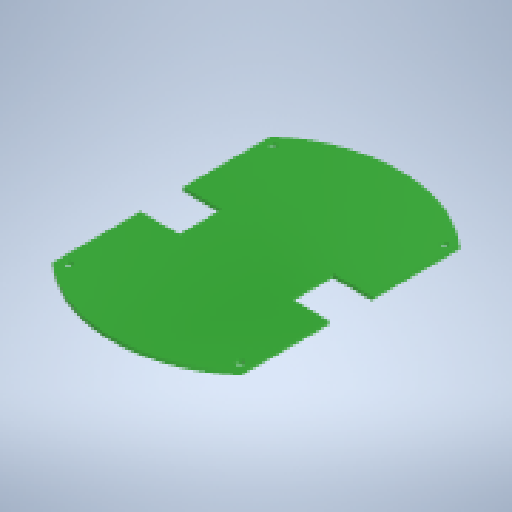
# Autodesk Inventor part: BaseBoard3
Saved by Autodesk Inventor 2025.3 (Build 293356000, 356)
## iProperties
Created: 2025-05-29
Part Number: BaseBoard3
Material: 一般
Document SubType Name: Modeling
Designer: yamashita1
Density: 1 g/cm^3
Appearance: 滑らか - 濃い深緑
Author: yamashita1
Autodesk Inventor part; units mm, degrees
ref_plane "YZ Plane" through (0, 0, 0) normal (1, 0, 0) x (0, 1, 0)
ref_plane "XZ Plane" through (0, 0, 0) normal (0, 1, 0) x (-1, 0, 0)
ref_plane "XY Plane" through (0, 0, 0) normal (0, 0, 1) x (1, 0, 0)
sketch "スケッチ1" plane through (0, 0, 0) normal (0, 0, 1) x (1, 0, 0)
  circle A0 centre (0, 0) radius 65 construction
  line L0 (-42.5, 65) -> (42.5, 65) construction
  line L1 (42.5, 65) -> (42.5, -65) construction
  line L2 (42.5, -65) -> (-42.5, -65) construction
  line L3 (-42.5, -65) -> (-42.5, 65) construction
  arc A1 (42.5, 49.1808) -> (-42.5, 49.1808) centre (0, 0) ccw
  line L4 (-42.5, 49.1808) -> (-42.5, -49.1808)
  line L5 (42.5, 49.1808) -> (42.5, -49.1808)
  arc A2 (-42.5, -49.1808) -> (42.5, -49.1808) centre (0, 0) ccw
  point P0 (0, 65)
  dimension "d0" = 130
  dimension "d1" = 85
  constraints: 14 end point, 9 point on circle, 4 point on line, 3 centre point, 3 parallel, 2 tangent, 1 coincident, 1 concentric, 1 horizontal, 1 midpoint, 1 perpendicular, 1 vertical, 1 vertical alignment
  measures "d0" diameter of A0
  measures "d1" distance of L1.end L2.end
extrude "基板" add sketch "スケッチ1" along normal blind 1.6
sketch "スケッチ4" plane through (0, 0, 1.6) normal (0, 0, 1) x (1, 0, 0)
  line L0 (0, -55.1622) -> (0, 55.1622) construction
  line L1 (42.5, -49.1808) -> (42.5, 49.1808) construction
  circle A0 centre (0, 0) radius 60 construction
  line L2 (0, 0) -> (36.3616, 43.334) construction
  line L3 (0, 0) -> (56.5685, 0) construction
  point P0 (38.5, -46.019)
  point P1 (-38.5, -46.019)
  point P2 (38.5673, 45.9627)
  point P3 (-38.5673, 45.9627)
  dimension "d27" = 4
  dimension "d29" = 120
  dimension "d30" = 50
  constraints: 6 end point, 2 coincident, 2 point on circle, 2 symmetric about line, 1 centre point, 1 equal length, 1 horizontal, 1 midpoint, 1 point on line, 1 vertical
  measures "d27" distance from line of L1 A0.end
  measures "d29" diameter of A0
  measures "d30" angle of L3 L2
hole "スペーサ取付穴" at (38.5, -46.019, 1.6) at (-38.5, -46.019, 1.6) at (38.5673, 45.9627, 1.6) at (-38.5673, 45.9627, 1.6) direction (0, 0, -1) diameter 3.2 end through all
sketch "スケッチ6" plane through (0, 0, 1.6) normal (0, 0, 1) x (1, 0, 0)
  line L0 (-42.5, 49.1808) -> (-42.5, -49.1808) projected
  line L1 (-42.5, 9.5) -> (-25, 9.5)
  line L2 (-25, 9.5) -> (-25, -9.5)
  line L3 (-25, -9.5) -> (-42.5, -9.5)
  line L4 (-42.5, -9.5) -> (-42.5, 9.5)
  line L5 (42.5, 9.5) -> (25, 9.5)
  line L6 (25, 9.5) -> (25, -9.5)
  line L7 (25, -9.5) -> (42.5, -9.5)
  line L8 (42.5, -9.5) -> (42.5, 9.5)
  line L9 (42.5, -49.1808) -> (42.5, 49.1808) projected
  point P0 (0, 0)
  point P1 (-25, 0)
  dimension "d43" = 19
  dimension "d44" = 17.5
  constraints: 16 end point, 4 parallel, 3 point on line, 2 collinear, 2 horizontal, 2 perpendicular, 1 horizontal alignment, 1 midpoint
  measures "d43" distance of L1.end L2.end
  measures "d44" distance of L1.start L1.end
extrude "モータ用切欠き" cut sketch "スケッチ6" against normal through all
fillet "フィレット1" radius 1.5 4 edges at (-25, 9.5, 0.8) (-25, -9.5, 0.8) (25, 9.5, 0.8) (25, -9.5, 0.8)
